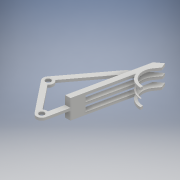
# Autodesk Inventor part: 三角塊4
Saved by Autodesk Inventor 2017 (Build 210142000, 142)
## iProperties
Part Number: 三角塊4
Material: 一般
Document SubType Name: Modeling
Designer: user
Density: 1 g/cm^3
Appearance: 預設
Author: user
Autodesk Inventor part; units mm, degrees
ref_plane "YZ Plane" through (0, 0, 0) normal (1, 0, 0) x (0, 1, 0)
ref_plane "XZ Plane" through (0, 0, 0) normal (0, 1, 0) x (-1, 0, 0)
sketch "草圖1" plane through (0, 0, 0) normal (0, 0, 1) x (1, 0, 0)
  line L0 (1.20216, 1.598378) -> (16.319323, 21.697976)
  line L1 (17.521484, 23.296354) -> (10.290449, -10.457794)
  line L2 (9.871501, -12.413423) -> (0, 0)
  line L3 (15.923106, 24.498514) -> (-1.598378, 1.20216)
  line L4 (-1.565375, -1.24483) -> (8.306126, -13.658253)
  line L5 (19.477112, 22.877407) -> (11.82713, -12.83237)
  arc A0 (10.290449, -10.457794) -> (8.626671, -10.848048) centre (9.871501, -12.413423) ccw
  arc A1 (8.306126, -13.658253) -> (11.82713, -12.83237) centre (9.871501, -12.413423) ccw
  arc A2 (19.477112, 22.877407) -> (15.923106, 24.498514) centre (17.521484, 23.296354) ccw
  arc A3 (16.319323, 21.697976) -> (17.102536, 21.340726) centre (17.521484, 23.296354) ccw
  arc A4 (-1.598378, 1.20216) -> (-1.565375, -1.24483) centre (0, 0) ccw
  arc A5 (1.24483, -1.565375) -> (1.20216, 1.598378) centre (0, 0) ccw
  dimension "d0" = 36.52
  dimension "d1" = 29.15
  dimension "d2" = 15.86
  constraints: 12 end point, 12 point on circle, 6 centre point, 6 tangent, 3 coincident, 3 point on line
  measures "d0" distance of L1.start L2.start
  measures "d1" distance of L2.end L1.start
  measures "d2" distance of L2.start L2.end
extrude "擠出1" add sketch "草圖1" along normal blind 1
sketch "草圖2" plane through (0, 0, 0) normal (0, 0, -1) x (-1, 0, 0)
  circle A0 centre (0, 0) radius 0.75
  dimension "d8" = 1.5
  constraints: 1 centre point, 1 coincident
  measures "d8" diameter of A0
extrude "擠出2" add sketch "草圖2" along normal blind 1
sketch "草圖3" plane through (0, 0, 0) normal (0, 0, -1) x (-1, 0, 0)
  arc A0 (-11.82713, -12.83237) -> (-8.306126, -13.658253) centre (-9.871501, -12.413423) ccw
  circle A1 centre (-9.871501, -12.413423) radius 1
  arc A2 (-15.923106, 24.498514) -> (-19.477112, 22.877407) centre (-17.521484, 23.296354) ccw
  circle A3 centre (-17.521484, 23.296354) radius 1
  point P0 (0, 0)
  dimension "d11" = 2
  dimension "d12" = 2
  constraints: 2 centre point, 2 coincident
  measures "d11" diameter of A3
  measures "d12" diameter of A1
extrude "擠出3" cut sketch "草圖3" against normal blind 1
sketch "草圖4" plane through (0, 0, 1) normal (0, 0, 1) x (1, 0, 0)
  circle A0 centre (0, 0) radius 1
  dimension "d15" = 2
  constraints: 1 centre point, 1 coincident
  measures "d15" diameter of A0
extrude "擠出4" cut sketch "草圖4" against normal blind 10
ref_plane "工作平面1" through (0, 0, 0.5) normal (0, 0, 1) x (1, 0, 0)
sketch "草圖5" plane through (0, 0, 0.5) normal (0, 0, 1) x (1, 0, 0)
  line L0 (11.82713, -12.83237) -> (19.477112, 22.877407)
  arc A0 (19.764563, 21.493066) -> (23.609175, 13.296354) centre (23.609175, 18.296354) ccw
  circle A1 centre (17.521484, 23.296354) radius 1
  arc A2 (18.995641, 22.132408) -> (23.609175, 12.296354) centre (23.609175, 18.296354) ccw
  arc A3 (19.764563, 21.493066) -> (17.521484, 23.296354) centre (18.657909, 22.413225) ccw
  line L1 (23.609175, 13.296354) -> (23.609175, 12.296354)
  arc A4 (18.995641, 22.132408) -> (18.311091, 22.682741) centre (18.657909, 22.413225) ccw
  line L2 (17.521484, 23.296354) -> (18.311091, 22.682741)
  point P0 (0, 0)
  dimension "d18" = 10
  dimension "d20" = 5
  dimension "d21" = 1
  constraints: 8 point on circle, 4 centre point, 4 end point, 3 tangent
  measures "d18" diameter of A0
  measures "d20" vertical distance of A0.centre L2.start
  measures "d21" radial gap between concentric circles of A0 A2
revolve "迴轉1" add sketch "草圖5" angle 9.4 mid plane about axis through (23.609175, 13.296354, 0.5) along (0, -1, 0) picked at (17.90254, 23.23482) contours A2 A4 A1 A3 A0 L0 | L0 A0 L1 A2 | L2 A3 A1
sketch "草圖6" plane through (0, 0, 0.5) normal (0, 0, 1) x (1, 0, 0)
  line L0 (17.521484, 23.296354) -> (17.541954, 23.296354)
  line L1 (15.923106, 24.498514) -> (-1.598378, 1.20216)
  ellipse E0 centre (18.674558, 22.413225) end of major axis (18.674558, 23.852454) minor radius 1.434389 (18.373214, 23.820335) -> (17.541954, 23.296354) ccw
  line L2 (11.593712, 18.742204) -> (17.541954, 23.296354)
  arc A0 (19.496644, 23.610585) -> (17.494598, 23.260097) centre (18.674558, 22.413225) ccw
  arc A1 (19.496644, 23.610585) -> (15.923106, 24.498514) centre (17.521484, 23.296354) ccw
  point P0 (0, 0)
  constraints: 6 point on circle, 3 point on line, 2 centre point, 2 coincident, 2 end point, 1 other
extrude "擠出5" cut sketch "草圖6" along normal mid plane 10 contours A0 L2 L1 A1
sketch "草圖8" plane through (0, 0, 0.5) normal (0, 0, 1) x (1, 0, 0)
  line L0 (16.735106, 22.678608) -> (11.593712, 18.742204)
  line L1 (16.735106, 22.678608) -> (20.206166, 25.336154)
  line L2 (20.206166, 25.336154) -> (21.018758, 23.273436)
  ellipse E0 centre (18.674558, 22.413225) end of major axis (18.674558, 23.852454) minor radius 1.434389 (19.777491, 21.493066) -> (19.499743, 23.590444) ccw
  line L3 (21.018758, 23.273436) -> (19.851898, 21.591106)
  line L4 (19.851898, 21.591106) -> (12.756322, 16.960653)
  line L5 (1.20216, 1.598378) -> (16.319323, 21.697976)
  line L6 (11.593712, 18.742204) -> (12.756322, 16.960653)
  point P0 (0, 0)
  constraints: 10 end point, 1 perpendicular, 1 point on line, 3 other
extrude "擠出6" add sketch "草圖8" along normal mid plane 1
sketch "草圖9" plane through (0, 0, 1) normal (0, 0, 1) x (1, 0, 0)
  line L0 (11.82713, -12.83237) -> (19.095857, 21.097727)
  line L1 (14.576164, 0) -> (12.518579, 0)
  line L2 (12.518579, 0) -> (11.469308, -4.897952)
  line L3 (11.469308, -4.897952) -> (13.526893, -4.897952)
  line L4 (14.576164, 0) -> (13.526893, -4.897952)
  point P0 (0, 0)
  constraints: 8 end point, 2 parallel, 2 point on line, 1 collinear, 1 horizontal
extrude "擠出7" add sketch "草圖9" along normal blind 2.3
sketch "草圖11" plane through (0, 0, 3.3) normal (0, 0, 1) x (1, 0, 0)
  line L0 (14.576164, 0) -> (19.095857, 21.097727)
  line L1 (16.718062, 19.546017) -> (12.530786, 0)
  line L2 (13.526893, -4.897952) -> (14.576164, 0)
  line L3 (11.469308, -4.897952) -> (13.526893, -4.897952)
  line L4 (12.518579, 0) -> (11.469308, -4.897952)
  ellipse E0 centre (23.609175, 18.296354) end of major axis (23.609175, 13.296354) minor radius 4.983187 (19.777491, 21.493066) -> (23.609175, 13.296354) ccw
  ellipse E1 centre (23.609175, 18.296354) end of major axis (23.609175, 12.296354) minor radius 5.979824 (18.032029, 16.131822) -> (23.609175, 12.296354) ccw
  line L5 (23.609175, 13.296354) -> (23.609175, 12.296354)
  line L6 (16.718062, 19.546017) -> (17.517467, 23.277606)
  line L7 (11.593712, 18.742204) -> (20.206166, 25.336154)
  line L8 (21.018758, 23.273436) -> (20.206166, 25.336154)
  line L9 (20.206166, 25.336154) -> (21.018758, 23.273436)
  line L10 (21.018758, 23.273436) -> (19.777491, 21.493066)
  arc A0 (18.025357, 16.10068) -> (23.609175, 12.296354) centre (23.609175, 18.296354) ccw
  arc A1 (19.836327, 21.577455) -> (23.609175, 13.296354) centre (23.609175, 18.296354) ccw
  line L11 (23.609175, 13.296354) -> (23.609175, 12.296354)
  line L12 (20.206166, 25.336154) -> (17.517467, 23.277606)
  line L13 (12.756322, 16.960653) -> (16.718062, 19.546017)
  line L14 (10.290449, -10.457794) -> (16.718062, 19.546017)
  line L15 (16.718062, 19.546017) -> (11.469308, -4.897952)
  line L16 (13.526893, -4.897952) -> (11.481515, -4.897952)
  line L17 (11.469308, -4.897952) -> (13.526893, -4.897952)
  line L18 (13.526893, -4.897952) -> (18.025357, 16.10068)
  point P0 (0, 0)
  constraints: 18 end point, 4 point on circle, 3 point on line, 2 centre point, 2 coincident, 2 collinear, 1 horizontal, 1 vertical, 5 other
sketch "草圖11 outline for 擠出8" plane through (0, 0, 3.3) normal (0, 0, 1) x (1, 0, 0)
  line L0 (13.526893, -4.897952) -> (18.025357, 16.10068)
  line L1 (11.469308, -4.897952) -> (13.526893, -4.897952)
  line L2 (16.718062, 19.546017) -> (11.469308, -4.897952)
  line L3 (17.517467, 23.277606) -> (16.718062, 19.546017)
  line L4 (20.206166, 25.336154) -> (17.517467, 23.277606)
  line L5 (21.018758, 23.273436) -> (20.206166, 25.336154)
  line L6 (19.836327, 21.577455) -> (21.018758, 23.273436)
  arc A0 (23.609175, 13.296354) -> (19.836327, 21.577455) centre (23.609175, 18.296354) cw
  line L7 (23.609175, 12.296354) -> (23.609175, 13.296354)
  spline S0 degree 2 poles (18.032029, 16.131822) (19.510608, 12.296354) (23.609175, 12.296354) knots 0 0 0 1 1 1 weights 1 0.8248501 1
  line L8 (18.025357, 16.10068) -> (18.032029, 16.131822)
extrude "擠出8" add sketch "草圖11 outline for 擠出8" along normal blind 1
mirror "鏡射1" about plane through (0, 0, 0.5) normal (0, 0, 1) of "擠出8", "擠出7"
sketch "草圖12" plane through (0, 0, 0.5) normal (0, 0, 1) x (1, 0, 0)
  ellipse E0 centre (23.609175, 18.296354) end of major axis (23.609175, 13.296354) minor radius 4.983187 (19.777491, 21.493066) -> (23.609175, 13.296354) ccw
  line L0 (19.851898, 21.591106) -> (21.018758, 23.273436)
  line L1 (19.095857, 21.097727) -> (19.851898, 21.591106)
  line L2 (19.851898, 21.591106) -> (19.777491, 21.493066)
  line L3 (19.38552, 21.803658) -> (19.447146, 21.884858)
  line L4 (19.447146, 21.884858) -> (20.79834, 23.832954)
  line L5 (21.018758, 23.273436) -> (20.206166, 25.336154)
  line L6 (23.609175, 12.296354) -> (23.609175, 13.296354)
  line L7 (23.609175, 13.296354) -> (23.609175, 12.796354)
  spline S0 degree 5 poles (23.609175, 12.796296) (22.36611, 12.796205) (21.123215, 13.149796) (20.014498, 13.857213) (18.328076, 15.812862) (17.909063, 18.360813) (18.074623, 19.663579) (18.594533, 20.845424) (19.385489, 21.803684) knots 0 0 0 0 0 0 0.50010037 0.50010037 0.50010037 1 1 1 1 1 1
  point P0 (0, 0)
  dimension "d31" = 0.5
  constraints: 8 end point, 1 collinear, 1 parallel, 1 point on line, 5 other
  measures "d31" distance between parallel lines of L0 L4
extrude "擠出9" cut sketch "草圖12" along normal mid plane 1
